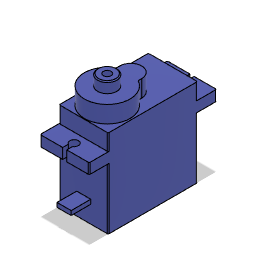
WisselWisselaarAssembly (Autodesk Fusion 360 archive; units mm, degrees)
design "Servo"
Autodesk Fusion 360 part; units mm, degrees
sketch "Body" plane through (0, 0, 0) normal (0, 1, 0) x (1, 0, 0) in component "servo"
  line L0 (6.25, -11.375) -> (-6.25, -11.375)
  line L1 (-6.25, -11.375) -> (-6.25, 11.375)
  line L2 (-6.25, 11.375) -> (6.25, 11.375)
  line L3 (6.25, 11.375) -> (6.25, -11.375)
  line L4 (6.25, -11.375) -> (-6.25, 11.375) construction
  line L5 (-6.25, -11.375) -> (6.25, 11.375) construction
  dimension "d6" = 12.5
  dimension "d7" = 22.75
  dimension "d52" = 0
  dimension "d53" = 0
  dimension "d54" = 0
  constraint perpendicular L0 L1
  constraint parallel L0 L2
  constraint parallel L1 L3
  constraint horizontal L0
  constraint coincident L4 origin
  constraint coincident L5 origin
  measures "d6" distance of L1.end L2.end
  measures "d7" distance of L0.end L1.end
extrude "Extrude1" add sketch "Body" along normal blind 22.35 makes body 1 in component "servo"
sketch "Tab" plane through (0, 0, 11.375) normal (0, 0, 1) x (1, 0, 0) in component "servo"
  line L0 (-6.25, 0) -> (6.25, 0)
  line L1 (6.25, 0) -> (6.25, 22.35)
  line L2 (6.25, 22.35) -> (-6.25, 22.35)
  line L3 (-6.25, 22.35) -> (-6.25, 0)
  line L4 (-6.25, 18.2) -> (6.25, 18.2)
  line L5 (6.25, 18.2) -> (6.25, 15.55)
  line L6 (6.25, 15.55) -> (-6.25, 15.55)
  line L7 (-6.25, 15.55) -> (-6.25, 18.2)
  dimension "d10" = 4.15
  dimension "d11" = 2.65
  constraint horizontal L4
  constraint vertical L5
  constraint horizontal L6
  constraint vertical L7
  constraint coincident L1 L5.end
  constraint coincident L3 L4.start
  measures "d10" distance of L1.end L4.end
  measures "d11" distance of L4.end L5.end
extrude "Extrude2" add sketch "Tab" along normal blind 4.85 contours L1 L3 L4 L5 L6 L7 bodies 1 in component "servo"
hole "Hole1" at (0, 18.2, 13.8) direction (0, -1, 0) diameter 2.2 end through all bodies 1 in component "servo"
fillet "Fillet1" radius 0.25 2 edges at (6.25, 16.875, 16.225) (-6.25, 16.875, 16.225) on bodies 1 in component "servo"
sketch "Notch" plane through (0, 0, 16.225) normal (0, 0, 1) x (1, 0, 0) in component "servo"
  line L0 (-6, 18.2) -> (-6, 15.55)
  line L1 (-6, 15.55) -> (6, 15.55)
  line L2 (6, 15.55) -> (6, 18.2)
  line L3 (6, 18.2) -> (-6, 18.2)
  line L4 (-0.525, 18.2) -> (0.525, 18.2)
  line L5 (0.525, 18.2) -> (0.525, 15.55)
  line L6 (0.525, 15.55) -> (-0.525, 15.55)
  line L7 (-0.525, 15.55) -> (-0.525, 18.2)
  dimension "d20" = 1.05
  constraint collinear L3 L4
  constraint collinear L1 L6
  constraint parallel L5 L7
  measures "d20" distance of L4.start L4.end
extrude "Extrude3" cut sketch "Notch" along normal up to surface contours L1 L3 L4 L5 L6 L7 end surface at (0.0548, 17.3167, 14.8986) on bodies 1 bodies 1 in component "servo"
mirror "Mirror1" about plane through (0, 0, 0) normal (0, 0, 1) of "Extrude2", "Hole1", "Fillet1", "Extrude3" in component "servo"
sketch "Bump" plane through (0, 22.35, 0) normal (0, 1, 0) x (-1, 0, 0) in component "servo"
  line L0 (-6.25, -11.375) -> (6.25, -11.375)
  line L1 (6.25, -11.375) -> (6.25, 11.375)
  line L2 (6.25, 11.375) -> (-6.25, 11.375)
  line L3 (-6.25, 11.375) -> (-6.25, -11.375)
  line L4 (-2.8, -0.625) -> (-2.8, 0.2671)
  line L5 (2.8, 0.2671) -> (2.8, -0.625)
  arc A0 (-2.8, -0.625) -> (2.8, -0.625) centre (0, -0.625) ccw
  arc A1 (2.8, 0.2671) -> (-2.8, 0.2671) centre (0, 5.375) ccw
  dimension "d23" = 11.65
  dimension "d24" = 6
  dimension "d25" = 5.6
  dimension "d26" = 6
  dimension "d27" = 6.25
  dimension "d28" = 6.25
  constraint tangent L4 A0
  constraint vertical L4
  constraint tangent L5 A0
  measures "d23" diameter of A1
  measures "d24" distance of L2 A1.centre
  measures "d25" diameter of A0
  measures "d26" distance of A1.centre A0.centre
  measures "d27" distance of L3 A1.centre
  measures "d28" distance of L3 A0.centre
extrude "Extrude4" add sketch "Bump" along normal blind 4.3 contours L4 L5 A0 A1 bodies 1 in component "servo"
fillet "Fillet2" radius 0.25 8 edges at (6.25, 7.775, 11.375) (6.25, 20.275, 11.375) (-6.25, 20.275, 11.375) (-6.25, 7.775, 11.375) (6.25, 7.775, -11.375) (6.25, 20.275, -11.375) (-6.25, 20.275, -11.375) (-6.25, 7.775, -11.375) on bodies 1 in component "servo"
sketch "Wire" plane through (0, 0, 11.375) normal (0, 0, 1) x (1, 0, 0) in component "servo"
  line L0 (-6, 15.55) -> (-6, 0)
  line L1 (-6, 0) -> (6, 0)
  line L2 (6, 0) -> (6, 15.55)
  line L3 (6, 15.55) -> (-6, 15.55)
  line L4 (-1.8, 5.5) -> (1.8, 5.5)
  line L5 (1.8, 5.5) -> (1.8, 4.4)
  line L6 (1.8, 4.4) -> (-1.8, 4.4)
  line L7 (-1.8, 4.4) -> (-1.8, 5.5)
  dimension "d32" = 1.1
  dimension "d33" = 3.6
  constraint horizontal L4
  constraint vertical L5
  constraint horizontal L6
  constraint vertical L7
  measures "d32" distance of L4.start L6.end
  measures "d33" distance of L4.start L4.end
  measures "d34" distance of L1 L4.end
extrude "Extrude5" add sketch "Wire" along normal blind 5 contours L4 L5 L6 L7 bodies 1 in component "servo"
hole "Hole2" at (0, 26.65, 5.375) direction (0, -1, 0) diameter 4.92 depth 15 tip angle 180 bodies 1 in component "servo"
cylinder "CylinderPrimitive1" add diameter 4.92 height 2.72 placed x (1, 0, 0) y (0, 0, -1) z (0, 1, 0) at (0, 26.65, 5.375) separate body makes body 2 in component "splined-drive"
extrude "Extrude1'" add 1 faces at (-0.4548, 26.65, 5.9711) along direction (0, -1, 0) blind 15 on bodies 2 bodies 2 in component "splined-drive"
hole "Hole1'" at (0, 29.37, 5.375) direction (0, -1, 0) diameter 1.95 depth 5 tip angle 180 bodies 2 in component "splined-drive"
chamfer "Chamfer1" distance 0.25 angle 45 1 edges at (-2.2935, 29.37, 6.2646) on bodies 2 in component "splined-drive"
component "servo" placed x (1, 0, 0) y (0, 1, 0) z (0, 0, 1) at (0, 0, 0)
component "splined-drive" placed x (1, 0, 0) y (0, 1, 0) z (0, 0, 1) at (0, 0, 0)

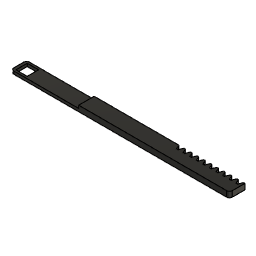
design "WisselArm"
Autodesk Fusion 360 part; units mm, degrees
sketch "Sketch1" plane through (0, 0, 0) normal (0, 0, 1) x (1, 0, 0)
  line L0 (1, 0) -> (78.5, 0)
  line L1 (79.5, 1) -> (79.5, 5.5)
  line L2 (0, 4.5) -> (0, 1)
  line L3 (79.5, 5.5) -> (79.068, 5.5)
  line L4 (79.068, 5.5) -> (78.8314, 5.1243)
  line L5 (79.068, 5.5) -> (79.4858, 5.5) construction
  line L6 (78.8314, 5.1243) -> (78.4223, 4.0004)
  line L7 (78.4223, 4.0004) -> (77.7903, 4.0004)
  line L8 (77.7903, 4.0004) -> (77.3821, 5.1219)
  line L9 (77.1447, 5.5) -> (77.3813, 5.1243)
  line L10 (77.3813, 5.1243) -> (77.7903, 4.0004)
  line L11 (77.7903, 4.0004) -> (78.4223, 4.0004)
  line L12 (74.8035, 5.5) -> (74.3857, 5.5) construction
  line L13 (74.3715, 5.5) -> (74.8035, 5.5)
  line L14 (76.4903, 5.1243) -> (76.0812, 4.0004)
  line L15 (75.0401, 5.1243) -> (75.4492, 4.0004)
  line L16 (76.0812, 4.0004) -> (76.4894, 5.1219)
  line L17 (75.4492, 4.0004) -> (76.0812, 4.0004)
  line L18 (76.0812, 4.0004) -> (75.4492, 4.0004)
  line L19 (76.7269, 5.5) -> (76.4903, 5.1243)
  line L20 (74.8035, 5.5) -> (75.0401, 5.1243)
  line L21 (70.7527, 4.0004) -> (71.3847, 4.0004)
  line L22 (69.6751, 5.5) -> (70.1071, 5.5)
  line L23 (74.3715, 5.5) -> (74.7894, 5.5) construction
  line L24 (71.3847, 4.0004) -> (70.7527, 4.0004)
  line L25 (70.3437, 5.1243) -> (69.1411, 5.1243) construction
  line L26 (72.4482, 5.5) -> (72.0304, 5.5) construction
  line L27 (74.3715, 5.5) -> (74.1349, 5.1243)
  line L28 (70.1071, 5.5) -> (69.6893, 5.5) construction
  line L29 (73.7259, 4.0004) -> (73.0939, 4.0004)
  line L30 (70.1071, 5.5) -> (70.3437, 5.1243)
  line L31 (72.0304, 5.5) -> (71.7938, 5.1243)
  line L32 (72.2393, 5.5) -> (72.2393, 4)
  line L33 (74.8035, 5.5) -> (74.3715, 5.5)
  line L34 (73.4099, 4.0004) -> (73.4099, 5.5)
  line L35 (72.0304, 5.5) -> (72.4482, 5.5) construction
  line L36 (71.3847, 4.0004) -> (71.7929, 5.1219)
  line L37 (71.0687, 4.0004) -> (71.0687, 5.5)
  line L38 (72.2393, 5.5) -> (72.2393, 4)
  line L39 (72.6848, 5.1243) -> (73.0939, 4.0004)
  line L40 (70.3437, 5.1243) -> (70.7527, 4.0004)
  line L41 (71.7938, 5.1243) -> (71.3847, 4.0004)
  line L42 (73.0939, 4.0004) -> (72.6857, 5.1219)
  line L43 (72.4482, 5.5) -> (72.6848, 5.1243)
  line L44 (74.1349, 5.1243) -> (73.7259, 4.0004)
  line L45 (73.0939, 4.0004) -> (73.7259, 4.0004)
  line L46 (69.8982, 5.5) -> (69.8982, 4)
  line L47 (61.374, 4.0004) -> (62.006, 4.0004)
  line L48 (65.4248, 5.5) -> (64.9928, 5.5)
  line L49 (64.9928, 5.5) -> (65.4106, 5.5) construction
  line L50 (62.8606, 5.5) -> (62.8606, 4)
  line L51 (60.2963, 5.5) -> (60.7283, 5.5)
  line L52 (63.0695, 5.5) -> (62.6517, 5.5) construction
  line L53 (60.9649, 5.1243) -> (59.7624, 5.1243) construction
  line L54 (65.6614, 5.1243) -> (64.4589, 5.1243) construction
  line L55 (70.1213, 5.5) -> (69.6893, 5.5)
  line L56 (66.7025, 4.0004) -> (67.1107, 5.1219)
  line L57 (67.7659, 5.5) -> (68.0025, 5.1243)
  line L58 (62.4151, 5.1243) -> (62.006, 4.0004)
  line L59 (64.7562, 5.1243) -> (65.9587, 5.1243) construction
  line L60 (62.006, 4.0004) -> (61.374, 4.0004)
  line L61 (65.2088, 5.5) -> (65.2088, 4)
  line L62 (64.9928, 5.5) -> (64.7562, 5.1243)
  line L63 (61.69, 4.0004) -> (61.69, 5.5)
  line L64 (62.6517, 5.5) -> (63.0695, 5.5) construction
  line L65 (60.7283, 5.5) -> (60.3105, 5.5) construction
  line L66 (63.7151, 4.0004) -> (63.3069, 5.1219)
  line L67 (64.0311, 4.0004) -> (64.0311, 5.5)
  line L68 (62.006, 4.0004) -> (62.4142, 5.1219)
  line L69 (64.9928, 5.5) -> (65.4248, 5.5)
  line L70 (65.4248, 5.5) -> (65.007, 5.5) construction
  line L71 (60.9649, 5.1243) -> (61.374, 4.0004)
  line L72 (69.0436, 4.0004) -> (68.4116, 4.0004)
  line L73 (63.7151, 4.0004) -> (64.3471, 4.0004)
  line L74 (68.0025, 5.1243) -> (68.4116, 4.0004)
  line L75 (68.4116, 4.0004) -> (68.0034, 5.1219)
  line L76 (62.6517, 5.5) -> (62.4151, 5.1243)
  line L77 (65.6614, 5.1243) -> (66.0705, 4.0004)
  line L78 (69.6893, 5.5) -> (69.4527, 5.1243)
  line L79 (69.4527, 5.1243) -> (69.0436, 4.0004)
  line L80 (60.7283, 5.5) -> (60.9649, 5.1243)
  line L81 (63.3061, 5.1243) -> (63.7151, 4.0004)
  line L82 (69.8982, 5.5) -> (69.8982, 4)
  line L83 (62.8606, 5.5) -> (62.8606, 4)
  line L84 (66.0705, 4.0004) -> (66.7025, 4.0004)
  line L85 (66.7025, 4.0004) -> (66.0705, 4.0004)
  line L86 (65.2088, 5.5) -> (65.2088, 4)
  line L87 (67.1115, 5.1243) -> (66.7025, 4.0004)
  line L88 (67.3481, 5.5) -> (67.1115, 5.1243)
  line L89 (64.7562, 5.1243) -> (64.3471, 4.0004)
  line L90 (65.4248, 5.5) -> (65.6614, 5.1243)
  line L91 (69.6893, 5.5) -> (70.1071, 5.5) construction
  line L92 (66.3865, 4.0004) -> (66.3865, 5.5)
  line L93 (68.7276, 4.0004) -> (68.7276, 5.5)
  line L94 (63.0695, 5.5) -> (63.3061, 5.1243)
  line L95 (67.557, 5.5) -> (67.557, 4)
  line L96 (67.7659, 5.5) -> (67.3481, 5.5) construction
  line L97 (64.3471, 4.0004) -> (63.7151, 4.0004)
  line L98 (67.3481, 5.5) -> (67.7659, 5.5) construction
  line L99 (68.4116, 4.0004) -> (69.0436, 4.0004)
  line L100 (67.557, 5.5) -> (67.557, 4)
  line L101 (60.5123, 5.5) -> (60.5123, 4)
  line L102 (57.9552, 5.5) -> (57.7186, 5.1243)
  line L103 (57.7186, 5.1243) -> (57.3095, 4.0004)
  line L104 (58.6096, 5.1243) -> (59.0187, 4.0004)
  line L105 (59.0187, 4.0004) -> (58.6105, 5.1219)
  line L106 (57.3095, 4.0004) -> (56.6775, 4.0004)
  line L107 (56.9935, 4.0004) -> (56.9935, 5.5)
  line L108 (60.7283, 5.5) -> (60.2963, 5.5)
  line L109 (60.2963, 5.5) -> (60.0597, 5.1243)
  line L110 (58.1641, 5.5) -> (58.1641, 4)
  line L111 (60.2963, 5.5) -> (60.7142, 5.5) construction
  line L112 (59.6507, 4.0004) -> (59.0187, 4.0004)
  line L113 (56.2685, 5.1243) -> (56.6775, 4.0004)
  line L114 (59.0187, 4.0004) -> (59.6507, 4.0004)
  line L115 (60.0597, 5.1243) -> (61.2623, 5.1243) construction
  line L116 (59.3347, 4.0004) -> (59.3347, 5.5)
  line L117 (57.3095, 4.0004) -> (57.7177, 5.1219)
  line L118 (60.5123, 5.5) -> (60.5123, 4)
  line L119 (56.6775, 4.0004) -> (57.3095, 4.0004)
  line L120 (56.0319, 5.5) -> (56.2685, 5.1243)
  line L121 (60.0597, 5.1243) -> (59.6507, 4.0004)
  line L122 (58.1641, 5.5) -> (58.1641, 4)
  line L123 (58.373, 5.5) -> (58.6096, 5.1243)
  line L124 (55.5999, 5.5) -> (1, 5.5)
  line L125 (55.5999, 5.5) -> (56.0319, 5.5)
  line L126 (56.0319, 5.5) -> (56.2685, 5.1243)
  line L127 (76.7269, 5.5) -> (77.1447, 5.5)
  line L128 (56.0319, 5.5) -> (56.2685, 5.1243)
  line L129 (57.9552, 5.5) -> (58.373, 5.5)
  line L130 (62.6517, 5.5) -> (63.0695, 5.5)
  line L131 (67.3481, 5.5) -> (67.7659, 5.5)
  line L132 (72.0304, 5.5) -> (72.4482, 5.5)
  arc A0 (1, 5.5) -> (0, 4.5) centre (1, 4.5) ccw
  arc A1 (0, 1) -> (1, 0) centre (1, 1) ccw
  arc A2 (78.5, 0) -> (79.5, 1) centre (78.5, 1) ccw
  point P0 (79.5, 0)
  point P1 (0, 5.5)
  dimension "d1" = 79.5
  dimension "d2" = 5.5
  dimension "d30" = 1
  dimension "d33" = 122.2
  dimension "d34" = 110
  dimension "d35" = 0.444
  dimension "d36" = 1.1239
  dimension "d37" = 0.632
  dimension "d38" = 1.1215
  dimension "d39" = 0.444
  dimension "d40" = 0.4178
  dimension "d41" = 110
  dimension "d42" = 110
  dimension "d43" = 122.2
  dimension "d44" = 167.8
  dimension "d45" = 0.3757
  dimension "d46" = 1.196
  dimension "d47" = 0.632
  dimension "d48" = 1.7091
  dimension "d49" = 110
  dimension "d50" = 110
  dimension "d51" = 1.1239
  dimension "d52" = 0.444
  dimension "d53" = 0.4178
  constraint horizontal L0
  constraint vertical L1
  constraint vertical L2
  constraint perpendicular L1 L3
  constraint horizontal L5
  constraint midpoint L28 L46.start
  constraint perpendicular L25 L46
  constraint symmetric L1.end L46 L51.start
  constraint symmetric L3.end L46 L51.end
  constraint symmetric L4.end L46 L53.start
  constraint symmetric L5.end L46 L65.end
  constraint symmetric L6.end L46 L47.start
  constraint symmetric L7.end L46 L47.end
  constraint symmetric L8.end L46 L68.end
  constraint symmetric L9.start L46 L52.end
  constraint symmetric L9.end L46 L58.start
  constraint symmetric L19.start L46 L52.start
  constraint symmetric L14.end L46 L66.start
  constraint symmetric L12.start L46 L48.end
  constraint symmetric L13.start L46 L48.start
  constraint symmetric L12.end L46 L49.end
  constraint symmetric L15.end L46 L73.end
  constraint symmetric L14.start L46 L81.start
  constraint symmetric L15.start L46 L59.start
  constraint symmetric L16.end L46 L66.end
  constraint symmetric L39.start L46 L87.start
  constraint symmetric L42.end L46 L56.end
  constraint symmetric L23.end L46 L70.end
  constraint symmetric L27.end L46 L54.start
  constraint symmetric L29.start L46 L77.end
  constraint symmetric L32.start L46 L95.start
  constraint symmetric L32.end L46 L95.end
  constraint symmetric L29.end L46 L56.start
  constraint symmetric L21.start L46 L72.start
  constraint symmetric L34.start L46 L92.start
  constraint symmetric L26.start L46 L88.start
  constraint symmetric L26.end L46 L57.start
  constraint symmetric L36.end L46 L75.end
  constraint symmetric L31.end L46 L57.end
  constraint symmetric L21.end L46 L72.end
  constraint symmetric L37.end L46 L93.end
  constraint symmetric L34.end L46 L92.end
  constraint symmetric L25.start L46 L78.end
  constraint symmetric L22.end L46 L28.end
  constraint symmetric L22.start L46 L55.start
  constraint symmetric L28.end L46 L22.end
  constraint symmetric L37.start L46 L93.start
  constraint symmetric L82.start L46 L46.start
  constraint symmetric L82.end L46 L46.end
  constraint midpoint L51 L101.start
  constraint perpendicular L51 L101
  constraint symmetric L67.end L101 L107.end
  constraint symmetric L47.end L101 L104.end
  constraint symmetric L67.start L101 L107.start
  constraint symmetric L66.start L101 L103.end
  constraint symmetric L48.end L101 L120.start
  constraint symmetric L73.end L101 L106.end
  constraint symmetric L81.start L101 L102.end
  constraint symmetric L50.end L101 L110.end
  constraint symmetric L66.end L101 L117.end
  constraint symmetric L47.start L101 L112.start
  constraint symmetric L50.start L101 L110.start
  constraint symmetric L52.start L101 L102.start
  constraint symmetric L53.start L101 L109.end
  constraint symmetric L51.start L101 L51.end
  constraint symmetric L65.end L101 L111.end
  constraint symmetric L51.end L101 L51.start
  constraint symmetric L52.end L101 L123.start
  constraint symmetric L48.start L101 L124.start
  constraint symmetric L63.end L101 L116.end
  constraint symmetric L63.start L101 L116.start
  constraint symmetric L68.end L101 L105.end
  constraint symmetric L53.end L101 L115.end
  constraint symmetric L58.start L101 L104.start
  constraint symmetric L118.start L101 L101.start
  constraint symmetric L118.end L101 L101.end
  constraint perpendicular L2 L124
  constraint parallel L124 L125
  constraint horizontal L127
  constraint horizontal L129
  constraint parallel L64 L130
  constraint parallel L98 L131
  constraint parallel L35 L132
  constraint coincident P1 L2
  constraint coincident P1 L124
  constraint tangent L2 A0
  constraint tangent L124 A0
  constraint coincident origin L0
  constraint coincident origin L2
  constraint tangent L0 A1
  constraint tangent L2 A1
  constraint equal A0 A1
  constraint coincident P0 L0
  constraint coincident P0 L1
  constraint tangent L0 A2
  constraint tangent L1 A2
  constraint equal A0 A2
  measures "d1" distance of origin P0
  measures "d2" distance of origin P1
  measures "d30" radius of A0
  measures "d33" angle of L125 L126 L32.end
  measures "d34" angle of L113 L124
  measures "d35" distance of L113.start L120.start
  measures "d36" vertical distance of L113.start L106.end
  measures "d37" distance of L103.end L106.end
  measures "d38" vertical distance of L103.end L117.end
  measures "d39" distance of L102.end L102.start
  measures "d40" distance of L102.start L123.start
  measures "d41" angle of L103 L119
  measures "d42" angle of L113 L119
  measures "d43" angle of L123 L129
  measures "d44" angle of L105 L123
  measures "d45" vertical distance of L104.start L123.start
  measures "d46" distance of L104.start L104.end
  measures "d47" distance of L104.end L112.start
  measures "d48" distance of L103.end L104.end
  measures "d49" angle of L104 L112
  measures "d50" angle of L114 L121
  measures "d51" vertical distance of L112.start L109.end
  measures "d52" distance of L109.end L51.start
  measures "d53" distance of L65.end L51.end
extrude "Extrude2" add sketch "Sketch1" along normal blind 2
sketch "Sketch2" plane through (0, 0, 2) normal (0, 0, 1) x (-1, 0, 0)
  line L0 (-71.7938, -5.1243) -> (-71.3847, -4.0004)
  line L1 (-71.3847, -4.0004) -> (-70.7527, -4.0004)
  line L2 (-70.7527, -4.0004) -> (-70.3437, -5.1243)
  line L3 (-70.3437, -5.1243) -> (-70.1071, -5.5)
  line L4 (-70.1071, -5.5) -> (-69.6893, -5.5)
  line L5 (-69.6893, -5.5) -> (-69.4527, -5.1243)
  line L6 (-69.4527, -5.1243) -> (-69.0436, -4.0004)
  line L7 (-69.0436, -4.0004) -> (-68.4116, -4.0004)
  line L8 (-68.4116, -4.0004) -> (-68.0025, -5.1243)
  line L9 (-68.0025, -5.1243) -> (-67.7659, -5.5)
  line L10 (-67.7659, -5.5) -> (-67.3481, -5.5)
  line L11 (-67.3481, -5.5) -> (-67.1115, -5.1243)
  line L12 (-67.1115, -5.1243) -> (-66.7025, -4.0004)
  line L13 (-66.7025, -4.0004) -> (-66.0705, -4.0004)
  line L14 (-66.0705, -4.0004) -> (-65.6614, -5.1243)
  line L15 (-65.6614, -5.1243) -> (-65.4248, -5.5)
  line L16 (-65.4248, -5.5) -> (-64.9928, -5.5)
  line L17 (-64.9928, -5.5) -> (-64.7562, -5.1243)
  line L18 (-64.7562, -5.1243) -> (-64.3471, -4.0004)
  line L19 (-64.3471, -4.0004) -> (-63.7151, -4.0004)
  line L20 (-63.7151, -4.0004) -> (-63.3061, -5.1243)
  line L21 (-63.3061, -5.1243) -> (-63.0695, -5.5)
  line L22 (-63.0695, -5.5) -> (-62.6517, -5.5)
  line L23 (-62.6517, -5.5) -> (-62.4151, -5.1243)
  line L24 (-62.4151, -5.1243) -> (-62.006, -4.0004)
  line L25 (-62.006, -4.0004) -> (-61.374, -4.0004)
  line L26 (-61.374, -4.0004) -> (-60.9649, -5.1243)
  line L27 (-60.9649, -5.1243) -> (-60.7283, -5.5)
  line L28 (-60.7283, -5.5) -> (-60.2963, -5.5)
  line L29 (-60.2963, -5.5) -> (-60.0597, -5.1243)
  line L30 (-60.0597, -5.1243) -> (-59.6507, -4.0004)
  line L31 (-59.6507, -4.0004) -> (-59.0187, -4.0004)
  line L32 (-59.0187, -4.0004) -> (-58.6096, -5.1243)
  line L33 (-58.6096, -5.1243) -> (-58.373, -5.5)
  line L34 (-58.373, -5.5) -> (-57.9552, -5.5)
  line L35 (-57.9552, -5.5) -> (-57.7186, -5.1243)
  line L36 (-57.7186, -5.1243) -> (-57.3095, -4.0004)
  line L37 (-57.3095, -4.0004) -> (-56.6775, -4.0004)
  line L38 (-56.6775, -4.0004) -> (-56.2685, -5.1243)
  line L39 (-56.2685, -5.1243) -> (-56.0319, -5.5)
  line L40 (-56.0319, -5.5) -> (-1, -5.5)
  line L41 (0, -4.5) -> (0, -1)
  line L42 (-1, 0) -> (-78.5, 0)
  line L43 (-79.5, -1) -> (-79.5, -5.5)
  line L44 (-79.5, -5.5) -> (-79.068, -5.5)
  line L45 (-79.068, -5.5) -> (-78.8314, -5.1243)
  line L46 (-78.8314, -5.1243) -> (-78.4223, -4.0004)
  line L47 (-78.4223, -4.0004) -> (-77.7903, -4.0004)
  line L48 (-77.7903, -4.0004) -> (-77.3813, -5.1243)
  line L49 (-77.3813, -5.1243) -> (-77.1447, -5.5)
  line L50 (-77.1447, -5.5) -> (-76.7269, -5.5)
  line L51 (-76.7269, -5.5) -> (-76.4903, -5.1243)
  line L52 (-76.4903, -5.1243) -> (-76.0812, -4.0004)
  line L53 (-76.0812, -4.0004) -> (-75.4492, -4.0004)
  line L54 (-75.4492, -4.0004) -> (-75.0401, -5.1243)
  line L55 (-75.0401, -5.1243) -> (-74.8035, -5.5)
  line L56 (-74.8035, -5.5) -> (-74.3715, -5.5)
  line L57 (-74.3715, -5.5) -> (-74.1349, -5.1243)
  line L58 (-74.1349, -5.1243) -> (-73.7259, -4.0004)
  line L59 (-73.7259, -4.0004) -> (-73.0939, -4.0004)
  line L60 (-73.0939, -4.0004) -> (-72.6848, -5.1243)
  line L61 (-72.6848, -5.1243) -> (-72.4482, -5.5)
  line L62 (-72.4482, -5.5) -> (-72.0304, -5.5)
  line L63 (-72.0304, -5.5) -> (-71.7938, -5.1243)
  line L64 (-3, -4.75) -> (-7, -4.75)
  line L65 (-7, -4.75) -> (-7, -0.75)
  line L66 (-7, -0.75) -> (-3, -0.75)
  line L67 (-3, -0.75) -> (-3, -4.75)
  arc A0 (-1, -5.5) -> (0, -4.5) centre (-1, -4.5) ccw
  arc A1 (0, -1) -> (-1, 0) centre (-1, -1) ccw
  arc A2 (-78.5, 0) -> (-79.5, -1) centre (-78.5, -1) ccw
  dimension "d22" = 4
  dimension "d23" = 4
  dimension "d26" = 0.75
  dimension "d32" = 5.5
  dimension "d63" = 3
  constraint horizontal L64
  constraint vertical L65
  constraint horizontal L66
  constraint vertical L67
  measures "d22" distance of L64.start L64.end
  measures "d23" distance of L64.start L66.end
  measures "d26" distance of L40 L64
  measures "d32" distance of L40 L42
  measures "d63" distance of L41 L67
extrude "Extrude3" cut sketch "Sketch2" against normal blind 2 contours L64 L65 L66 L67
sketch "Sketch3" plane through (0, 0, 2) normal (0, 0, 1) x (-1, 0, 0)
  line L0 (-7, -4.75) -> (-7, -0.75)
  line L1 (-7, -0.75) -> (-3, -0.75)
  line L2 (-3, -0.75) -> (-3, -4.75)
  line L3 (-3, -4.75) -> (-7, -4.75)
  line L4 (-56.0319, -5.5) -> (-1, -5.5)
  arc A0 (-1, -5.5) -> (0, -4.5) centre (-1, -4.5) ccw
  line L5 (0, -4.5) -> (0, -1)
  arc A1 (0, -1) -> (-1, 0) centre (-1, -1) ccw
  line L6 (-1, 0) -> (-78.5, 0)
  arc A2 (-78.5, 0) -> (-79.5, -1) centre (-78.5, -1) ccw
  line L7 (-79.5, -1) -> (-79.5, -5.5)
  line L8 (-79.5, -5.5) -> (-79.068, -5.5)
  line L9 (-79.068, -5.5) -> (-78.8314, -5.1243)
  line L10 (-78.8314, -5.1243) -> (-78.4223, -4.0004)
  line L11 (-78.4223, -4.0004) -> (-77.7903, -4.0004)
  line L12 (-77.7903, -4.0004) -> (-77.3813, -5.1243)
  line L13 (-77.3813, -5.1243) -> (-77.1447, -5.5)
  line L14 (-77.1447, -5.5) -> (-76.7269, -5.5)
  line L15 (-76.7269, -5.5) -> (-76.4903, -5.1243)
  line L16 (-76.4903, -5.1243) -> (-76.0812, -4.0004)
  line L17 (-76.0812, -4.0004) -> (-75.4492, -4.0004)
  line L18 (-75.4492, -4.0004) -> (-75.0401, -5.1243)
  line L19 (-75.0401, -5.1243) -> (-74.8035, -5.5)
  line L20 (-74.8035, -5.5) -> (-74.3715, -5.5)
  line L21 (-74.3715, -5.5) -> (-74.1349, -5.1243)
  line L22 (-74.1349, -5.1243) -> (-73.7259, -4.0004)
  line L23 (-73.7259, -4.0004) -> (-73.0939, -4.0004)
  line L24 (-73.0939, -4.0004) -> (-72.6848, -5.1243)
  line L25 (-72.6848, -5.1243) -> (-72.4482, -5.5)
  line L26 (-72.4482, -5.5) -> (-72.0304, -5.5)
  line L27 (-72.0304, -5.5) -> (-71.7938, -5.1243)
  line L28 (-71.7938, -5.1243) -> (-71.3847, -4.0004)
  line L29 (-71.3847, -4.0004) -> (-70.7527, -4.0004)
  line L30 (-70.7527, -4.0004) -> (-70.3437, -5.1243)
  line L31 (-70.3437, -5.1243) -> (-70.1071, -5.5)
  line L32 (-70.1071, -5.5) -> (-69.6893, -5.5)
  line L33 (-69.6893, -5.5) -> (-69.4527, -5.1243)
  line L34 (-69.4527, -5.1243) -> (-69.0436, -4.0004)
  line L35 (-69.0436, -4.0004) -> (-68.4116, -4.0004)
  line L36 (-68.4116, -4.0004) -> (-68.0025, -5.1243)
  line L37 (-68.0025, -5.1243) -> (-67.7659, -5.5)
  line L38 (-67.7659, -5.5) -> (-67.3481, -5.5)
  line L39 (-67.3481, -5.5) -> (-67.1115, -5.1243)
  line L40 (-67.1115, -5.1243) -> (-66.7025, -4.0004)
  line L41 (-66.7025, -4.0004) -> (-66.0705, -4.0004)
  line L42 (-66.0705, -4.0004) -> (-65.6614, -5.1243)
  line L43 (-65.6614, -5.1243) -> (-65.4248, -5.5)
  line L44 (-65.4248, -5.5) -> (-64.9928, -5.5)
  line L45 (-64.9928, -5.5) -> (-64.7562, -5.1243)
  line L46 (-64.7562, -5.1243) -> (-64.3471, -4.0004)
  line L47 (-64.3471, -4.0004) -> (-63.7151, -4.0004)
  line L48 (-63.7151, -4.0004) -> (-63.3061, -5.1243)
  line L49 (-63.3061, -5.1243) -> (-63.0695, -5.5)
  line L50 (-63.0695, -5.5) -> (-62.6517, -5.5)
  line L51 (-62.6517, -5.5) -> (-62.4151, -5.1243)
  line L52 (-62.4151, -5.1243) -> (-62.006, -4.0004)
  line L53 (-62.006, -4.0004) -> (-61.374, -4.0004)
  line L54 (-61.374, -4.0004) -> (-60.9649, -5.1243)
  line L55 (-60.9649, -5.1243) -> (-60.7283, -5.5)
  line L56 (-60.7283, -5.5) -> (-60.2963, -5.5)
  line L57 (-60.2963, -5.5) -> (-60.0597, -5.1243)
  line L58 (-60.0597, -5.1243) -> (-59.6507, -4.0004)
  line L59 (-59.6507, -4.0004) -> (-59.0187, -4.0004)
  line L60 (-59.0187, -4.0004) -> (-58.6096, -5.1243)
  line L61 (-58.6096, -5.1243) -> (-58.373, -5.5)
  line L62 (-58.373, -5.5) -> (-57.9552, -5.5)
  line L63 (-57.9552, -5.5) -> (-57.7186, -5.1243)
  line L64 (-57.7186, -5.1243) -> (-57.3095, -4.0004)
  line L65 (-57.3095, -4.0004) -> (-56.6775, -4.0004)
  line L66 (-56.6775, -4.0004) -> (-56.2685, -5.1243)
  line L67 (-56.2685, -5.1243) -> (-56.0319, -5.5)
  line L68 (-2, -5.5) -> (0, -5.5)
  line L69 (0, -5.5) -> (0, 0)
  line L70 (0, 0) -> (-2, 0)
  line L71 (-2, 0) -> (-2, -5.5)
  constraint horizontal L68
  constraint vertical L69
  constraint horizontal L70
  constraint vertical L71
  constraint coincident L69.end L70.start
  constraint coincident L4 L68.start
extrude "Extrude4" cut sketch "Sketch3" against normal up to surface (2 mm away) contours L4 A0 L5 A1 L6 L68 L69 L70 L71
fillet "Fillet1" radius 1 1 edges at (2, 5.5, 1)
fillet "Fillet2" radius 1 1 edges at (2, 0, 1)
sketch "Sketch4" plane through (0, 0, 2) normal (0, 0, 1) x (-1, 0, 0)
  arc A0 (-2, -1) -> (-3, 0) centre (-3, -1) ccw
  line L0 (-3, 0) -> (-78.5, 0)
  arc A1 (-78.5, 0) -> (-79.5, -1) centre (-78.5, -1) ccw
  line L1 (-79.5, -1) -> (-79.5, -5.5)
  line L2 (-79.5, -5.5) -> (-79.068, -5.5)
  line L3 (-79.068, -5.5) -> (-78.8314, -5.1243)
  line L4 (-78.8314, -5.1243) -> (-78.4223, -4.0004)
  line L5 (-78.4223, -4.0004) -> (-77.7903, -4.0004)
  line L6 (-77.7903, -4.0004) -> (-77.3813, -5.1243)
  line L7 (-77.3813, -5.1243) -> (-77.1447, -5.5)
  line L8 (-77.1447, -5.5) -> (-76.7269, -5.5)
  line L9 (-76.7269, -5.5) -> (-76.4903, -5.1243)
  line L10 (-76.4903, -5.1243) -> (-76.0812, -4.0004)
  line L11 (-76.0812, -4.0004) -> (-75.4492, -4.0004)
  line L12 (-75.4492, -4.0004) -> (-75.0401, -5.1243)
  line L13 (-75.0401, -5.1243) -> (-74.8035, -5.5)
  line L14 (-74.8035, -5.5) -> (-74.3715, -5.5)
  line L15 (-74.3715, -5.5) -> (-74.1349, -5.1243)
  line L16 (-74.1349, -5.1243) -> (-73.7259, -4.0004)
  line L17 (-73.7259, -4.0004) -> (-73.0939, -4.0004)
  line L18 (-73.0939, -4.0004) -> (-72.6848, -5.1243)
  line L19 (-72.6848, -5.1243) -> (-72.4482, -5.5)
  line L20 (-72.4482, -5.5) -> (-72.0304, -5.5)
  line L21 (-72.0304, -5.5) -> (-71.7938, -5.1243)
  line L22 (-71.7938, -5.1243) -> (-71.3847, -4.0004)
  line L23 (-71.3847, -4.0004) -> (-70.7527, -4.0004)
  line L24 (-70.7527, -4.0004) -> (-70.3437, -5.1243)
  line L25 (-70.3437, -5.1243) -> (-70.1071, -5.5)
  line L26 (-70.1071, -5.5) -> (-69.6893, -5.5)
  line L27 (-69.6893, -5.5) -> (-69.4527, -5.1243)
  line L28 (-69.4527, -5.1243) -> (-69.0436, -4.0004)
  line L29 (-69.0436, -4.0004) -> (-68.4116, -4.0004)
  line L30 (-68.4116, -4.0004) -> (-68.0025, -5.1243)
  line L31 (-68.0025, -5.1243) -> (-67.7659, -5.5)
  line L32 (-67.7659, -5.5) -> (-67.3481, -5.5)
  line L33 (-67.3481, -5.5) -> (-67.1115, -5.1243)
  line L34 (-67.1115, -5.1243) -> (-66.7025, -4.0004)
  line L35 (-66.7025, -4.0004) -> (-66.0705, -4.0004)
  line L36 (-66.0705, -4.0004) -> (-65.6614, -5.1243)
  line L37 (-65.6614, -5.1243) -> (-65.4248, -5.5)
  line L38 (-65.4248, -5.5) -> (-64.9928, -5.5)
  line L39 (-64.9928, -5.5) -> (-64.7562, -5.1243)
  line L40 (-64.7562, -5.1243) -> (-64.3471, -4.0004)
  line L41 (-64.3471, -4.0004) -> (-63.7151, -4.0004)
  line L42 (-63.7151, -4.0004) -> (-63.3061, -5.1243)
  line L43 (-63.3061, -5.1243) -> (-63.0695, -5.5)
  line L44 (-63.0695, -5.5) -> (-62.6517, -5.5)
  line L45 (-62.6517, -5.5) -> (-62.4151, -5.1243)
  line L46 (-62.4151, -5.1243) -> (-62.006, -4.0004)
  line L47 (-62.006, -4.0004) -> (-61.374, -4.0004)
  line L48 (-61.374, -4.0004) -> (-60.9649, -5.1243)
  line L49 (-60.9649, -5.1243) -> (-60.7283, -5.5)
  line L50 (-60.7283, -5.5) -> (-60.2963, -5.5)
  line L51 (-60.2963, -5.5) -> (-60.0597, -5.1243)
  line L52 (-60.0597, -5.1243) -> (-59.6507, -4.0004)
  line L53 (-59.6507, -4.0004) -> (-59.0187, -4.0004)
  line L54 (-59.0187, -4.0004) -> (-58.6096, -5.1243)
  line L55 (-58.6096, -5.1243) -> (-58.373, -5.5)
  line L56 (-58.373, -5.5) -> (-57.9552, -5.5)
  line L57 (-57.9552, -5.5) -> (-57.7186, -5.1243)
  line L58 (-57.7186, -5.1243) -> (-57.3095, -4.0004)
  line L59 (-57.3095, -4.0004) -> (-56.6775, -4.0004)
  line L60 (-56.6775, -4.0004) -> (-56.2685, -5.1243)
  line L61 (-56.2685, -5.1243) -> (-56.0319, -5.5)
  line L62 (-56.0319, -5.5) -> (-3, -5.5)
  arc A2 (-3, -5.5) -> (-2, -4.5) centre (-3, -4.5) ccw
  line L63 (-2, -4.5) -> (-2, -1)
  line L64 (-7, -4.75) -> (-7, -0.75)
  line L65 (-7, -0.75) -> (-3, -0.75)
  line L66 (-3, -0.75) -> (-3, -4.75)
  line L67 (-3, -4.75) -> (-7, -4.75)
  line L68 (-2, 0) -> (-26, 0)
  line L69 (-26, 0) -> (-26, -5.5)
  line L70 (-26, -5.5) -> (-2, -5.5)
  line L71 (-2, -5.5) -> (-2, 0)
  dimension "d60" = 24
  constraint horizontal L68
  constraint vertical L69
  constraint horizontal L70
  constraint vertical L71
  constraint coincident L62 L69.end
  measures "d60" distance of L68.start L68.end
extrude "Extrude5" cut sketch "Sketch4" against normal blind 1 contours A0 L0 L62 A2 L63 L68 L69 L70 L71
equation "d26 = ( ( 5.5 - 4 ) / 2 ) * 1 mm"
